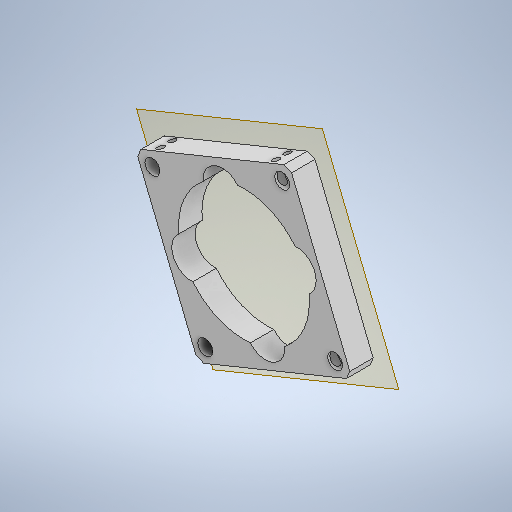
# Autodesk Inventor part: genera_ mount
Saved by Autodesk Inventor 2025.1 (Build 291241000, 241)
## iProperties
Created: 2024-11-20
Part Number: genera_ mount
Material: Ogólny
Document SubType Name: Modeling
Designer: PC
Density: 1 g/cm^3
Appearance: Domyślna
Author: PC
Autodesk Inventor part; units mm, degrees
ref_plane "YZ Plane" through (0, 0, 0) normal (1, 0, 0) x (0, 1, 0)
ref_plane "XZ Plane" through (0, 0, 0) normal (0, 1, 0) x (-1, 0, 0)
ref_plane "XY Plane" through (0, 0, 0) normal (0, 0, 1) x (1, 0, 0)
ref_plane "Płaszczyzna konstrukcyjna1" through (-33.6113, -84.498, -273.8281) normal (0, 0, 1) x (0.9260228, 0.3774677, 0)
sketch "Szkic1" plane through (-33.6113, -84.498, -273.8281) normal (0, 0, 1) x (0.9260228, 0.3774677, 0)
  circle A0 centre (63.0201, 65.5599) radius 3 projected
  circle A1 centre (3.0201, 65.5599) radius 3 projected
  circle A2 centre (3.0201, 5.5599) radius 3 projected
  circle A3 centre (63.0201, 5.5599) radius 3 projected
  line L0 (68.58, 2.54) -> (68.58, 68.58) projected
  line L1 (68.58, 68.58) -> (66.04, 71.12) projected
  line L2 (66.04, 71.12) -> (0, 71.12) projected
  line L3 (0, 71.12) -> (-2.54, 68.58) projected
  line L4 (-2.54, 68.58) -> (-2.54, 2.54) projected
  line L5 (0, 0) -> (66.04, 0) projected
  line L6 (-2.54, 2.54) -> (0, 0) projected
  line L7 (66.04, 0) -> (68.58, 2.54) projected
  arc A4 (13.76, 15.3185) -> (13.76, 55.8015) centre (33.1114, 35.56) ccw construction
  circle A5 centre (33.1114, 35.56) radius 28.0035
  circle A6 centre (3.0201, 65.5599) radius 3.2
  circle A7 centre (63.0201, 65.5599) radius 3.2
  circle A8 centre (63.0201, 5.5599) radius 3.2
  circle A9 centre (3.0201, 5.5599) radius 3.2
  circle A10 centre (33.1114, 59.938) radius 8.3317
  circle A11 centre (8.7334, 35.56) radius 8.3317
  circle A12 centre (33.1114, 11.182) radius 8.3317
  circle A13 centre (57.4894, 35.56) radius 8.3317
  point P0 (63.0201, 65.5599)
  dimension "d10" = 6.4
  dimension "d19" = 56.007
  dimension "d22" = 360
  constraints: 9 centre point, 5 coincident, 3 equal radius, 9 other
  measures "d10" diameter of A6
  measures "d19" diameter of A5
extrude "Wyciągnięcie proste1" add sketch "Szkic1" along normal blind 10 contours L7 L5 L6 L4 L3 L2 L1 L0
sketch "Szkic3" plane through (-60.4568, -18.6393, -263.8281) normal (-0.3774677, 0.9260228, 0) x (0.9260228, 0.3774677, 0)
  line L0 (6.2201, 0) -> (-0.1799, 0) construction
  line L1 (6.2201, 10) -> (-0.1799, 10) construction
  line L2 (66.2201, 0) -> (59.8201, 0) construction
  line L3 (66.2201, 10) -> (59.8201, 10) construction
  line L4 (6.2201, 10) -> (6.2201, 0) construction
  line L5 (66.04, 10) -> (0, 10) construction
  line L6 (33.02, 10) -> (33.02, 0) construction
  line L7 (66.04, 0) -> (0, 0) construction
  circle A0 centre (6.4201, 7.5) radius 1.5
  circle A1 centre (6.4201, 2.5) radius 1.5788
  line L8 (6.4201, 7.5) -> (6.4201, 2.5) construction
  line L9 (-2.54, 10) -> (-2.54, 0) construction
  circle A2 centre (59.6199, 7.5) radius 1.5
  circle A3 centre (59.6199, 2.5) radius 1.5788
  point P0 (63.0201, -263.8281)
  point P1 (6.4201, 5)
  point P2 (-2.54, 5)
  dimension "d11" = 3
  dimension "d12" = 5
  dimension "d13" = 0.2
  constraints: 6 end point, 4 centre point, 4 midpoint, 2 symmetric about line, 1 horizontal alignment, 1 perpendicular, 1 vertical, 2 other
  measures "d11" diameter of A0
  measures "d12" distance of L8.end L8.start
  measures "d13" distance between parallel lines of L4 L8
extrude "Wyciągnięcie proste3" cut sketch "Szkic3" against normal blind 15
pattern_circular "Szyk kołowy2" count 2 over 360 about axis through (-16.3721, -39.0702, -273.8281) along (0, 0, 1) of "Wyciągnięcie proste3"
